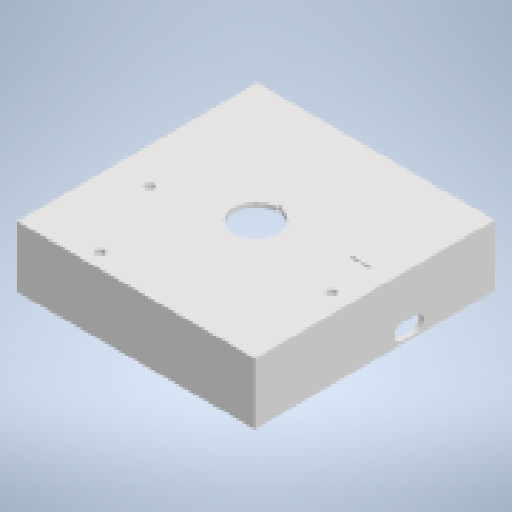
# Autodesk Inventor part: Parte inferior
Saved by Autodesk Inventor 2024 (Build 280153000, 153)
## iProperties
Created: 2023-07-04
Part Number: Parte inferior
Material: Generic
Document SubType Name: Modeling
Designer: Kleber
Density: 1 g/cm^3
Appearance: Default
Author: Kleber
Autodesk Inventor part; units mm, degrees
ref_plane "YZ Plane" through (0, 0, 0) normal (1, 0, 0) x (0, 1, 0)
ref_plane "XZ Plane" through (0, 0, 0) normal (0, 1, 0) x (-1, 0, 0)
ref_plane "XY Plane" through (0, 0, 0) normal (0, 0, 1) x (1, 0, 0)
sketch "Sketch1" plane through (0, 0, 0) normal (0, 1, 0) x (-1, 0, 0)
  line L0 (-48.611, 110.4452) -> (-48.611, 10.4452)
  line L1 (-48.611, 111.4452) -> (52.389, 111.4452)
  line L2 (52.389, 111.4452) -> (52.389, 9.4452)
  line L3 (52.389, 9.4452) -> (-48.611, 9.4452)
  line L4 (-48.611, 10.4452) -> (-48.611, 9.4452)
  line L5 (-48.611, 110.4452) -> (-48.611, 111.4452)
  line L6 (54.389, 7.4452) -> (54.389, 113.4452)
  line L7 (54.389, 113.4452) -> (-50.611, 113.4452)
  line L8 (-50.611, 113.4452) -> (-50.611, 110.4452)
  line L9 (-50.611, 110.4452) -> (-50.611, 10.4452)
  line L10 (-50.611, 10.4452) -> (-50.611, 7.4452)
  line L11 (-50.611, 7.4452) -> (54.389, 7.4452)
  point P0 (0, 0)
  dimension "d1" = 2
  constraints: 24 end point, 2 parallel, 2 perpendicular, 1 vertical, 5 other
  measures "d1" distance between parallel lines of L2 L6
extrude "Extrusion1" add sketch "Sketch1" along normal blind 25
sketch "Sketch2" plane through (0, 25, 0) normal (0, 1, 0) x (1, 0, 0)
  line L0 (-54.389, -7.4452) -> (-54.389, -113.4452) projected
  line L1 (50.611, -113.4452) -> (50.611, -7.4452) projected
  line L2 (-54.389, -113.4452) -> (50.611, -113.4452)
  line L3 (50.611, -113.4452) -> (50.611, -7.4452)
  line L4 (50.611, -7.4452) -> (-54.389, -7.4452)
  line L5 (-54.389, -7.4452) -> (-54.389, -113.4452)
  point P0 (0, 0)
  constraints: 8 end point, 2 parallel, 1 horizontal, 1 perpendicular
extrude "Extrusion2" add sketch "Sketch2" along normal blind 2
sketch "Sketch3" plane through (0, 25, 0) normal (0, -1, 0) x (1, 0, 0)
  line L0 (48.611, 9.4452) -> (48.611, 111.4452) projected
  line L1 (48.611, 111.4452) -> (-52.389, 111.4452) projected
  line L2 (-52.389, 111.4452) -> (-52.389, 9.4452) projected
  line L3 (-52.389, 9.4452) -> (48.611, 9.4452) projected
  line L4 (-52.389, 9.4452) -> (-43.389, 9.4452)
  line L5 (-43.389, 9.4452) -> (-43.389, 18.4452)
  line L6 (-43.389, 18.4452) -> (-52.389, 18.4452)
  line L7 (-52.389, 18.4452) -> (-52.389, 9.4452)
  line L8 (48.611, 9.4452) -> (39.611, 9.4452)
  line L9 (39.611, 9.4452) -> (39.611, 18.4452)
  line L10 (39.611, 18.4452) -> (48.611, 18.4452)
  line L11 (48.611, 18.4452) -> (48.611, 9.4452)
  line L12 (48.611, 111.4452) -> (39.611, 111.4452)
  line L13 (39.611, 111.4452) -> (39.611, 102.4452)
  line L14 (39.611, 102.4452) -> (48.611, 102.4452)
  line L15 (48.611, 102.4452) -> (48.611, 111.4452)
  line L16 (-52.389, 111.4452) -> (-43.389, 111.4452)
  line L17 (-43.389, 111.4452) -> (-43.389, 102.4452)
  line L18 (-43.389, 102.4452) -> (-52.389, 102.4452)
  line L19 (-52.389, 102.4452) -> (-52.389, 111.4452)
  point P0 (0, 0)
  dimension "d6" = 9
  dimension "d7" = 9
  dimension "d8" = 9
  dimension "d9" = 9
  dimension "d10" = 9
  dimension "d11" = 9
  dimension "d12" = 9
  constraints: 32 end point, 8 parallel, 4 horizontal, 4 perpendicular
  measures "d6" distance of L6.end L5.end
  measures "d7" distance of L5.end L4.end
  measures "d8" distance of L9.end L10.end
  measures "d9" distance of L14.end L13.end
  measures "d10" distance of L13.end L12.end
  measures "d11" distance of L17.end L18.end
  measures "d12" distance of L16.end L17.end
extrude "Extrusion3" add sketch "Sketch3" along normal blind 23.394 contours L3 L9 L10 L0 | L14 L13 L1 L0 | L3 L2 L6 L5 | L17 L18 L2 L1
sketch "Sketch4" plane through (0, 1.606, 0) normal (0, -1, 0) x (1, 0, 0)
  line L0 (-52.389, 9.4452) -> (-52.389, 18.4452) projected
  line L1 (-43.389, 9.4452) -> (-52.389, 9.4452) projected
  line L2 (-43.389, 9.4452) -> (-43.389, 18.4452) projected
  line L3 (-43.389, 18.4452) -> (-52.389, 18.4452) projected
  line L4 (-43.389, 102.4452) -> (-43.389, 111.4452) projected
  line L5 (-52.389, 111.4452) -> (-43.389, 111.4452) projected
  line L6 (-52.389, 102.4452) -> (-52.389, 111.4452) projected
  line L7 (-52.389, 102.4452) -> (-43.389, 102.4452) projected
  line L8 (48.611, 111.4452) -> (48.611, 102.4452) projected
  line L9 (39.611, 111.4452) -> (48.611, 111.4452) projected
  line L10 (39.611, 111.4452) -> (39.611, 102.4452) projected
  line L11 (39.611, 102.4452) -> (48.611, 102.4452) projected
  line L12 (39.611, 18.4452) -> (39.611, 9.4452) projected
  line L13 (48.611, 9.4452) -> (39.611, 9.4452) projected
  line L14 (48.611, 18.4452) -> (48.611, 9.4452) projected
  line L15 (48.611, 18.4452) -> (39.611, 18.4452) projected
  line L16 (-52.389, 102.4452) -> (-52.389, 18.4452) projected
  line L17 (39.611, 9.4452) -> (39.611, 18.4452) projected
  circle A0 centre (-47.889, 13.9452) radius 1.5
  circle A1 centre (-47.889, 106.9452) radius 1.5
  circle A2 centre (44.111, 106.9452) radius 1.5
  circle A3 centre (44.111, 13.9452) radius 1.5
  point P0 (0, 0)
  dimension "d15" = 3
  dimension "d16" = 3
  dimension "d17" = 3
  dimension "d18" = 3
  constraints: 4 centre point
  measures "d15" diameter of A0
  measures "d16" diameter of A1
  measures "d17" diameter of A2
  measures "d18" diameter of A3
extrude "Extrusion4" cut sketch "Sketch4" against normal blind 20 contours A0 | A1 | A2 | A3
sketch "Sketch5" plane through (50.611, 0, 113.4452) normal (1, 0, 0) x (0, 0, -1)
  line L0 (71.0695, 1.15) -> (65.3163, 1.15)
  line L1 (71.0695, 8.15) -> (65.3163, 8.15)
  arc A0 (65.3163, 8.15) -> (65.3163, 1.15) centre (65.3163, 4.65) ccw
  arc A1 (71.0695, 1.15) -> (71.0695, 8.15) centre (71.0695, 4.65) ccw
  line L2 (106, 0) -> (0, 0) projected
  point P0 (113.4452, 0)
  constraints: 4 end point, 4 point on circle, 2 centre point, 2 tangent, 1 horizontal, 1 parallel
extrude "Extrusion5" cut sketch "Sketch5" against normal blind 20
sketch "Sketch6" plane through (0, 27, 0) normal (0, 1, 0) x (1, 0, 0)
  line L0 (37.644, -52.7652) -> (37.644, -53.7652) projected
  line L1 (41.578, -53.7652) -> (41.578, -52.7652) projected
  line L2 (37.644, -53.7652) -> (41.578, -53.7652)
  line L3 (41.578, -53.7652) -> (41.578, -52.7652)
  line L4 (41.578, -52.7652) -> (37.644, -52.7652)
  line L5 (37.644, -52.7652) -> (37.644, -53.7652)
  point P0 (0, 0)
  constraints: 8 end point, 2 parallel, 1 horizontal, 1 perpendicular
extrude "Extrusion6" cut sketch "Sketch6" against normal blind 20
sketch "Sketch7" plane through (0, 27, 0) normal (0, 1, 0) x (1, 0, 0)
  circle A0 centre (-24.1564, -107.1543) radius 1.9651 projected
  circle A1 centre (-38.523, -70.7508) radius 1.9118 projected
  circle A2 centre (42.3862, -71.3336) radius 1.8923 projected
  line L0 (32.644, -52.7652) -> (32.644, -53.7652) projected
  line L1 (36.578, -53.7652) -> (36.578, -52.7652) projected
  line L2 (32.644, -53.7652) -> (36.578, -53.7652)
  line L3 (36.578, -53.7652) -> (36.578, -52.7652)
  line L4 (36.578, -52.7652) -> (32.644, -52.7652)
  line L5 (32.644, -52.7652) -> (32.644, -53.7652)
  point P0 (0, 0)
  constraints: 8 end point, 2 parallel, 1 horizontal, 1 perpendicular
extrude "Extrusion7" cut sketch "Sketch7" against normal blind 2
sketch "Sketch8" plane through (0, 27, 0) normal (0, 1, 0) x (1, 0, 0)
  circle A0 centre (42.3862, -71.3336) radius 1.8923 projected
  circle A1 centre (-24.1564, -107.1543) radius 1.9651 projected
  line L0 (32.644, -52.7652) -> (36.578, -52.7652) projected
  line L1 (36.578, -52.7652) -> (36.578, -53.7652) projected
  line L2 (36.578, -53.7652) -> (32.644, -53.7652) projected
  line L3 (32.644, -53.7652) -> (32.644, -52.7652) projected
  circle A2 centre (-38.523, -70.7508) radius 1.9118 projected
  line L4 (37.644, -52.7652) -> (41.578, -52.7652) projected
  line L5 (41.578, -52.7652) -> (41.578, -53.7652) projected
  line L6 (41.578, -53.7652) -> (37.644, -53.7652) projected
  line L7 (37.644, -53.7652) -> (37.644, -52.7652) projected
  line L8 (50.611, -113.4452) -> (50.611, -7.4452) projected
  line L9 (50.611, -7.4452) -> (-54.389, -7.4452) projected
  line L10 (-54.389, -7.4452) -> (-54.389, -113.4452) projected
  line L11 (-54.389, -113.4452) -> (50.611, -113.4452) projected
  line L12 (-54.389, -113.4452) -> (50.611, -113.4452) projected
  arc A3 (-2.7981, -50.4866) -> (-0.7981, -50.5048) centre (-1.889, -60.4452) ccw
  line L13 (-2.7981, -50.4866) -> (-2.7981, -49.4866)
  line L14 (-2.7981, -49.4866) -> (-0.7981, -49.4866)
  line L15 (-0.7981, -49.4866) -> (-0.7981, -50.5048)
  point P0 (0, 0)
  dimension "d37" = 1
  dimension "d38" = 2
  constraints: 6 end point, 2 perpendicular, 2 point on circle, 1 centre point, 1 vertical
  measures "d37" distance of L13.start L13.end
  measures "d38" distance of L13.end L14.end
extrude "Extrusion8" cut sketch "Sketch8" against normal blind 2 contours L13 L14 L15 A3
body "Solid1"
